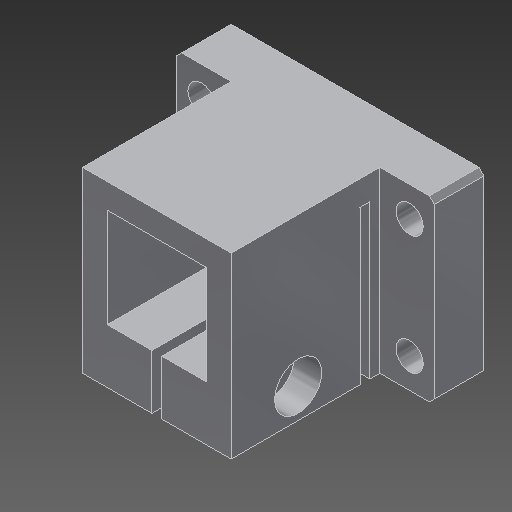
# Autodesk Inventor part: CLQAM20
Saved by Autodesk Inventor 2021.1 (Build 251245010, 245A)
## iProperties
Created: 2010-03-11
Part Number: CLQAM20
Document SubType Name: Modeling
Density: 1 g/cm^3
Material: MISUMI
Appearance: アルミニウム - フラット
Title: スタンドブラケット
Autodesk Inventor part; units mm, degrees
note: some values were not read from the file. Chosen so that the rebuilt part matches the saved one: direction of "穴2"; direction of "穴3".
ref_plane "YZ Plane" through (0, 0, 0) normal (1, 0, 0) x (0, 1, 0)
ref_plane "XZ Plane" through (0, 0, 0) normal (0, 1, 0) x (-1, 0, 0)
ref_plane "XY Plane" through (0, 0, 0) normal (0, 0, 1) x (1, 0, 0)
sketch "スケッチ1" plane through (0, 0, 0) normal (0, 0, 1) x (1, 0, 0)
  line L0 (-26, 18) -> (26, 18)
  line L1 (26, 18) -> (26, -18)
  line L2 (26, -18) -> (-26, -18)
  line L3 (-26, -18) -> (-26, 18)
  point P0 (0, 0)
  point P1 (0, -18)
  point P2 (-26, 0)
  dimension "d0" = 52
  dimension "d1" = 36
  constraints: 8 end point, 2 midpoint, 2 parallel, 1 horizontal, 1 horizontal alignment, 1 perpendicular, 1 vertical alignment
  measures "d0" distance of L1.end L2.end
  measures "d1" distance of L2.end L0.start
extrude "押し出し1" add sketch "スケッチ1" along normal blind 10
sketch "スケッチ2" plane through (0, 0, 10) normal (0, 0, 1) x (1, 0, 0)
  line L0 (-26, 18) -> (26, 18) projected
  line L1 (26, -18) -> (-26, -18) projected
  line L2 (-15, 18) -> (15, 18)
  line L3 (15, 18) -> (15, -18)
  line L4 (15, -18) -> (-15, -18)
  line L5 (-15, -18) -> (-15, 18)
  point P0 (0, 0)
  point P1 (0, -18)
  point P2 (0, -18)
  dimension "d4" = 30
  constraints: 8 end point, 2 midpoint, 2 parallel, 2 point on line, 1 coincident, 1 horizontal, 1 perpendicular
  measures "d4" distance between parallel lines of L3 L5
extrude "押し出し2" add sketch "スケッチ2" along normal blind 30
sketch "スケッチ3" plane through (0, 0, 40) normal (0, 0, 1) x (1, 0, 0)
  line L0 (15, -18) -> (-15, -18) projected
  line L1 (-10, 13) -> (10, 13)
  line L2 (10, 13) -> (10, -7)
  line L3 (10, -7) -> (-10, -7)
  line L4 (-10, -7) -> (-10, 13)
  point P0 (0, 0)
  point P1 (0, -7)
  dimension "d7" = 20
  dimension "d8" = 20
  dimension "d9" = 11
  constraints: 8 end point, 2 parallel, 1 horizontal, 1 midpoint, 1 perpendicular, 1 vertical alignment
  measures "d7" distance of L2.end L3.end
  measures "d8" distance of L3.end L1.start
  measures "d9" distance between parallel lines of L3 L0
extrude "押し出し3" cut sketch "スケッチ3" against normal through all
sketch "スケッチ4" plane through (0, 0, 10) normal (0, 0, 1) x (1, 0, 0)
  point P0 (0, 0)
  point P1 (-21, -12)
  dimension "d12" = 12
  dimension "d13" = 21
  measures "d12" vertical distance of point (-21, -12) point (0, 0)
  measures "d13" horizontal distance of point (-21, -12) point (0, 0)
hole "穴1" at (-21, -12, 10) direction (0, 0, -1) diameter 5.5 end through all
pattern_linear "矩形状パターン1" count 2 spacing 42 along (1, 0, 0) count 2 spacing 24 along (0, 1, 0) of "穴1"
sketch "スケッチ5" plane through (-26, -18, 0) normal (0, -1, 0) x (1, 0, 0)
  line L0 (41, 10) -> (41, 40) projected
  line L1 (41, 40) -> (11, 40) projected
  line L2 (11, 10) -> (11, 40) projected
  line L3 (52, 0) -> (0, 0) projected
  line L4 (11, 14) -> (41, 14)
  line L5 (41, 14) -> (41, 12)
  line L6 (41, 12) -> (11, 12)
  line L7 (11, 12) -> (11, 14)
  line L8 (25, 40) -> (27, 40)
  line L9 (27, 40) -> (27, 11.5)
  line L10 (27, 11.5) -> (25, 11.5)
  line L11 (25, 11.5) -> (25, 40)
  point P0 (26, 0)
  point P1 (26, 11.5)
  point P2 (26, 0)
  dimension "d27" = 12
  dimension "d28" = 2
  dimension "d29" = 2
  dimension "d30" = 0.5
  constraints: 16 end point, 4 parallel, 3 point on line, 2 horizontal, 2 midpoint, 2 perpendicular, 1 vertical alignment
  measures "d27" distance between parallel lines of L6 L3
  measures "d28" distance of L6.end L4.start
  measures "d29" distance of L9.end L10.end
  measures "d30" distance between parallel lines of L6 L10
extrude "押し出し4" cut sketch "スケッチ5" against normal up to surface (11 mm away) contours L6 L9 L4 L0 | L9 L10 L11 L6 | L6 L11 L4 L9 | L4 L11 L1 L9 | L6 L2 L4 L11
sketch "スケッチ6" plane through (-15, -7, 14) normal (0, -1, 0) x (1, 0, 0)
  line L0 (5, 0) -> (5, -2) projected
  line L1 (0, 0) -> (5, 0) projected
  line L2 (0, -2) -> (0, 0) projected
  line L3 (5, -2) -> (0, -2) projected
  line L4 (25, 0) -> (25, -2) projected
  line L5 (30, -2) -> (25, -2) projected
  line L6 (30, 0) -> (30, -2) projected
  line L7 (25, 0) -> (30, 0) projected
  point P0 (15, -14)
extrude "押し出し5" cut sketch "スケッチ6" against normal up to surface (20 mm away)
sketch "スケッチ7" plane through (15, -18, 10) normal (1, 0, 0) x (0, 0, -1)
  line L0 (-4, 0) -> (-30, 0) projected
  line L1 (10, 36) -> (10, 0) projected
  point P0 (10, 18)
  point P1 (-16.5, 6)
  dimension "d35" = 26.5
  dimension "d36" = 6
  measures "d35" distance from line of point (-16.5, 6) L1
  measures "d36" distance from line of point (-16.5, 6) L0
hole "穴2" at (15, -12, 26.5) direction (-1, 0, 0) diameter 5.5 end up to surface counterbore diameter 9.5 counterbore depth 5.5
sketch "スケッチ8" plane through (-15, -18, 10) normal (-1, 0, 0) x (0, 0, 1)
  circle A0 centre (16.5, 6) radius 2.75 projected
  point P0 (-10, 18)
hole "穴3" at (-15, -12, 26.5) direction (1, 0, 0) diameter 4.134 end up to surface thread size "M5x0.8" class "6H" standard "ANSI Metric M Profile"
chamfer "面取り1" distance 1 angle 45 4 edges at (-26, 18, 5) (-26, -18, 5) (26, 18, 5) (26, -18, 5)
equation "\"d8\" = d7"
